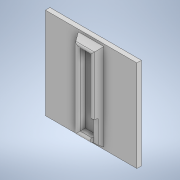
# Autodesk Inventor part: Weight_Plate
Saved by Autodesk Inventor 2021 (Build 250183000, 183)
## iProperties
Created: 2022-02-21
Part Number: Weight_Plate
Material: Generic
Document SubType Name: Modeling
Designer: aerts
Density: 1 g/cm^3
Appearance: Default
Author: aerts
Autodesk Inventor part; units mm, degrees
ref_plane "YZ Plane" through (0, 0, 0) normal (1, 0, 0) x (0, 1, 0)
ref_plane "XZ Plane" through (0, 0, 0) normal (0, 1, 0) x (-1, 0, 0)
ref_plane "XY Plane" through (0, 0, 0) normal (0, 0, 1) x (1, 0, 0)
sketch "Sketch1" plane through (0, 0, 0) normal (0, 0, 1) x (1, 0, 0)
  line L0 (0, 0) -> (100, 0)
  line L1 (100, 0) -> (100, 100)
  line L2 (100, 100) -> (0, 100)
  line L3 (0, 100) -> (0, 0)
  dimension "d0" = 100
  dimension "d1" = 100
  constraints: 8 end point, 2 parallel, 1 horizontal, 1 perpendicular
  measures "d0" distance of L1.end L2.end
  measures "d1" distance of L0.end L1.end
extrude "Extrusion1" add sketch "Sketch1" along normal blind 3
sketch "Sketch2" plane through (0, 0, 3) normal (0, 0, 1) x (1, 0, 0)
  line L0 (36, 97.5) -> (64, 97.5)
  line L1 (64, 97.5) -> (64, 2.5)
  line L2 (64, 2.5) -> (36, 2.5)
  line L3 (36, 2.5) -> (36, 97.5)
  line L4 (0, 0) -> (100, 0) projected
  line L5 (0, 100) -> (0, 0) projected
  dimension "d6" = 28
  dimension "d7" = 95
  dimension "d8" = 2.5
  dimension "d9" = 36
  constraints: 8 end point, 2 parallel, 1 horizontal, 1 perpendicular
  measures "d6" distance between parallel lines of L1 L3
  measures "d7" distance between parallel lines of L2 L0
  measures "d8" distance between parallel lines of L4 L2
  measures "d9" distance between parallel lines of L5 L3
extrude "Extrusion2" add sketch "Sketch2" along normal blind 13 draft -30
sketch "Sketch4" plane through (0, 0, 16) normal (0, 0, 1) x (1, 0, 0)
  line L0 (43.5056, 10.0056) -> (43.5056, 89.9944) projected
  line L1 (56.4944, 10.0056) -> (43.5056, 10.0056) projected
  line L2 (56.4944, 89.9944) -> (56.4944, 10.0056) projected
  line L3 (43.5056, 89.9944) -> (56.4944, 89.9944) projected
  point P0 (0, 0)
extrude "Extrusion3" cut sketch "Sketch4" against normal blind 13
sketch "Sketch5" plane through (0, 0, 0) normal (0, -1, 0) x (1, 0, 0)
  line L0 (56.4944, 16) -> (43.5056, 16) projected
  line L1 (43.5056, 16) -> (56.4944, 16) projected
  line L2 (56.2684, 16) -> (67.0318, 16)
  line L3 (67.0318, 16) -> (67.0318, 7)
  line L4 (67.0318, 7) -> (56.2684, 7)
  line L5 (56.2684, 7) -> (56.2684, 16)
  point P0 (0, 0)
  dimension "d14" = 9
  constraints: 8 end point, 2 parallel, 1 horizontal, 1 perpendicular, 1 point on line
  measures "d14" distance of L2.end L3.end
fillet "Fillet1" radius 2 4 edges at (50, 10.0056, 16) (56.4944, 50, 16) (43.5056, 50, 16) (50, 89.9944, 16)
extrude "Extrusion4" cut sketch "Sketch5" against normal blind 30
sketch "Sketch6" plane through (0, 0, 0) normal (0, 0, -1) x (-1, 0, 0)
  line L0 (-100, 100) -> (0, 100) projected
  line L1 (0, 0) -> (-100, 0) projected
  line L2 (-100, 100) -> (0, 100)
  line L3 (0, 100) -> (0, 0)
  line L4 (0, 0) -> (-100, 0)
  line L5 (-100, 0) -> (-100, 100)
  constraints: 8 end point, 2 parallel, 1 horizontal, 1 perpendicular
extrude "Extrusion5" add sketch "Sketch6" along normal blind 2
sketch "Sketch7" plane through (0, 0, -2) normal (0, 0, -1) x (-1, 0, 0)
  line L0 (-98, 98) -> (-2, 98)
  line L1 (-2, 98) -> (-2, 2)
  line L2 (-2, 2) -> (-98, 2)
  line L3 (-98, 2) -> (-98, 98)
  line L4 (0, 100) -> (-100, 100) projected
  line L5 (-100, 100) -> (-100, 0) projected
  line L6 (-100, 0) -> (0, 0) projected
  line L7 (0, 0) -> (0, 100) projected
  dimension "d19" = 2
  dimension "d20" = 2
  dimension "d21" = 2
  dimension "d22" = 2
  constraints: 8 end point, 2 parallel, 1 horizontal, 1 perpendicular
  measures "d19" distance between parallel lines of L4 L0
  measures "d20" distance between parallel lines of L5 L3
  measures "d21" distance between parallel lines of L6 L2
  measures "d22" distance between parallel lines of L7 L1
extrude "Extrusion6" cut sketch "Sketch7" against normal blind 2 contours L0 L1 L2 L3
body "Solid1"
